y_idler_bracket (Autodesk Fusion 360 design; units mm, degrees)
Autodesk Fusion 360 part; units mm, degrees
sketch "Sketch1" plane through (0, 0, 0) normal (0, 0, 1) x (1, 0, 0)
  line L0 (0, 13) -> (0, -13) construction
  circle A0 centre (0, 13) radius 1.7
  circle A1 centre (0, -13) radius 1.7
  line L1 (-15, 14.35) -> (15, 14.35)
  line L2 (15, 14.35) -> (15, -21.5)
  line L3 (15, -21.5) -> (-15, -21.5)
  line L4 (-15, -21.5) -> (-15, 14.35)
  line L5 (-15, 19.35) -> (15, 19.35)
  line L6 (15, 19.35) -> (15, 14.35)
  line L7 (-15, 14.35) -> (-15, 19.35)
  line L8 (-15, -18.5) -> (-12, -21.5)
  line L9 (15, -18.5) -> (12, -21.5)
  line L10 (15, 17) -> (-15, 17)
  line L11 (-0.7632, 11.3) -> (0.7632, 11.3)
  line L12 (-1.2042, 11.8) -> (1.2042, 11.8)
  line L13 (1.2704, 11.8704) -> (0.7632, 11.3)
  line L14 (-1.2704, 11.8704) -> (-0.7632, 11.3)
  line L15 (-0.7042, -14.7) -> (0.7042, -14.7)
  line L16 (1.2021, -14.2021) -> (0.7042, -14.7)
  line L17 (0, -13) -> (1.2021, -14.2021) construction
  line L18 (0, -13) -> (-1.2021, -14.2021) construction
  line L19 (-1.2021, -14.2021) -> (-0.7042, -14.7)
  circle A2 centre (0, -13) radius 2.25
  line L20 (-1.591, -14.591) -> (-0.932, -15.25)
  line L21 (1.591, -14.591) -> (0.932, -15.25)
  line L22 (0.932, -15.25) -> (-0.932, -15.25)
  line L23 (-1.4142, -14.75) -> (1.4142, -14.75)
  line L24 (-1.2042, -14.2) -> (1.2042, -14.2) construction
  circle A3 centre (0, 13) radius 2.25
  line L25 (1.0102, 10.75) -> (-1.0102, 10.75)
  line L26 (-1.6814, 11.5049) -> (-1.0102, 10.75)
  line L27 (1.6814, 11.5049) -> (1.0102, 10.75)
  point P0 (0, -13)
  point P1 (0, 13)
  point P2 (0, -15.25)
  point P3 (0, 10.75)
  dimension "d1" = 26
  dimension "d2" = 3.4
  dimension "d3" = 3.4
  dimension "d4" = 30
  dimension "d6" = 8.5
  dimension "d7" = 15
  dimension "d8" = 5
  dimension "d10" = 45
  dimension "d11" = 3
  dimension "d38" = 40.85
  dimension "d60" = 2.35
  dimension "d74" = 0.5
  dimension "d81" = 4.5
  dimension "d82" = 0.5
  dimension "d83" = 0.5
  dimension "d84" = 135
  dimension "d90" = 4.5
  constraint vertical L0
  constraint coincident L0.start A0.centre
  constraint midpoint origin L0
  constraint coincident P0 L0.end
  constraint horizontal L1
  constraint vertical L2
  constraint horizontal L3
  constraint vertical L4
  constraint horizontal L5
  constraint vertical L6
  constraint vertical L7
  constraint coincident L1.start L4.end
  constraint coincident L1.end L2.start
  constraint coincident L4 L8.start
  constraint coincident L3 L8.end
  constraint symmetric L0 L8.start L9.start
  constraint symmetric L0 L8.end L9.end
  constraint coincident P1 L0.start
  constraint coincident L6 L10.start
  constraint coincident L7 L10.end
  constraint horizontal L10
  constraint horizontal L11
  constraint tangent A0 L11
  constraint coincident A0 L12.start
  constraint coincident A0 L12.end
  constraint horizontal L12
  constraint coincident A0 L13.start
  constraint tangent A0 L13
  constraint coincident L11.end L13.end
  constraint coincident A0 L14.start
  constraint tangent A0 L14
  constraint coincident L11.start L14.end
  constraint horizontal L15
  constraint tangent A1 L15
  constraint coincident A1 L16.start
  constraint tangent A1 L16
  constraint coincident L15.end L16.end
  constraint perpendicular L16 L17
  constraint coincident L16.start L17.end
  constraint perpendicular L17 L18
  constraint coincident A1 L18.end
  constraint tangent A1 L19
  constraint coincident L15.start L19.end
  constraint perpendicular L18 L19
  constraint coincident A2 L20.start
  constraint tangent A2 L20
  constraint coincident A2 L21.start
  constraint tangent A2 L21
  constraint horizontal L22
  constraint coincident L20.end L22.end
  constraint tangent A2 L22
  constraint coincident A2 L23.start
  constraint coincident A2 L23.end
  constraint horizontal L23
  constraint coincident A1 L24.start
  constraint coincident A1 L24.end
  constraint horizontal L24
  constraint coincident A2 P2
  constraint coincident L0 P2
  constraint midpoint L22 P2
  constraint parallel L19 L20
  constraint concentric A0 A3
  constraint horizontal L25
  constraint coincident A3 P3
  constraint coincident L0 P3
  constraint midpoint L25 P3
  constraint coincident A3 L26.start
  constraint tangent A3 L26
  constraint coincident A3 L27.start
  constraint tangent A3 L27
  constraint coincident L25.start L27.end
  constraint coincident L25.end L26.end
  constraint parallel L14 L26
  constraint parallel L13 L27
  measures "d1" distance of L0.start P0
  measures "d2" diameter of A0
  measures "d3" diameter of A1
  measures "d4" distance of L1.start L1.end
  measures "d6" distance of P0 L3
  measures "d7" distance of P0 L2
  measures "d8" distance of L5.end L1.end
  measures "d10" angle of L3 L8
  measures "d11" distance of L3.end L8.end
  measures "d38" distance of L3.end L5.start
  measures "d60" distance of L5.end L10.start
  measures "d74" distance of L11 L12
  measures "d81" diameter of A2
  measures "d82" distance of L22 L23
  measures "d83" distance of L15 L24
  measures "d84" angle of L0 L17
  measures "d90" diameter of A3
extrude "Extrude1" add sketch "Sketch1" along normal blind 11.8 contours A0 L1 L12 | A0 L1 L11 L13 L14 A3 | A0 L11 L14 | A0 L12 | A0 L1 A3 | A0 L1 | A0 L11 L13 | L1 L2 L3 L4 L8 L9 A3 L25 L26 L27 | L1 L6 L7 L10 A3 | A3 L25 L26 | L5 L6 L7 L10 | A3 L25 L27 | A1 | A1 L15 L19 | A1 L15 L16 | A2 L23 | A2 L20 L22 | A2 L21 L22 | A2 L23
extrude "Extrude2" add sketch "Sketch1" along normal blind 54.6 contours A0 L1 A3 | A0 L1 | L1 L6 L7 L10 A3 | L5 L6 L7 L10
sketch "Sketch2" plane through (0, 14.35, 0) normal (0, -1, 0) x (1, 0, 0)
  line L0 (-15, 11.8) -> (15, 11.8)
  line L1 (15, 11.8) -> (15, 54.6)
  line L2 (15, 54.6) -> (-15, 54.6)
  line L3 (-15, 54.6) -> (-15, 11.8)
  circle A0 centre (0, 40) radius 1.6
  circle A1 centre (0, 40) radius 2.25
  dimension "d16" = 30
  dimension "d17" = 42.8
  dimension "d18" = 3.2
  dimension "d19" = 15
  dimension "d20" = 14.6
  dimension "d76" = 4.5
  constraint concentric A0 A1
  measures "d16" distance of L1.end L2.end
  measures "d17" distance of L0.end L1.end
  measures "d18" diameter of A0
  measures "d19" horizontal distance of L1.end A0.centre
  measures "d20" vertical distance of L1.end A0.centre
  measures "d76" diameter of A1
extrude "Extrude3" cut sketch "Sketch2" against normal blind 13 contours A0
extrude "Extrude6" cut sketch "Sketch1" along normal blind 6.8 contours A0 L1 L12 | A0 L11 L14 | A0 L12 | A0 L1 | A0 L11 L13 | A1 | A1 L15 L19 | A1 L15 L16
extrude "Extrude9" add sketch "Sketch1" against normal blind 4.2 contours L5 L6 L7 L10
extrude "Extrude11" cut sketch "Sketch2" against normal blind 5 contours A0 | A1
chamfer "Chamfer16" distance 0.625 angle 45 1 edges at (-2.0977, 19.35, 39.1864)
sketch "Sketch5" plane through (-15, 0, 0) normal (-1, 0, 0) x (0, -1, 0)
  line L0 (-17, 0) -> (18.5, 0)
  line L1 (18.5, 0) -> (18.5, 11.8)
  line L2 (18.5, 11.8) -> (-14.35, 11.8)
  line L3 (-14.35, 11.8) -> (-14.35, 54.6)
  line L4 (-14.35, 54.6) -> (-19.35, 54.6)
  line L5 (-19.35, 54.6) -> (-19.35, -4.2)
  line L6 (-19.35, -4.2) -> (-17, -4.2)
  line L7 (-17, -4.2) -> (-17, 0)
  circle A0 centre (-17, 0) radius 0.5
  dimension "d63" = 1
  constraint coincident L0.start L7.end
  measures "d63" diameter of A0
extrude "Extrude10" cut sketch "Sketch5" against normal blind 30 contours L0 L7 A0 | L0 L7 A0
chamfer "Chamfer1" distance 3 angle 45 2 edges at (15, 16.85, 54.6) (-15, 16.85, 54.6)
chamfer "Chamfer11" distance 20 angle 45 1 edges at (0, 14.35, 11.8)
chamfer "Chamfer2" distance 1 angle 45 12 edges at (-15, 14.35, 41.7) (-13.5, 14.35, 53.1) (0, 14.35, 54.6) (13.5, 14.35, 53.1) (15, 14.35, 41.7) (15, -12.075, 11.8) (13.5, -20, 11.8) (0, -21.5, 11.8) (-13.5, -20, 11.8) (-15, -12.075, 11.8) (-15, 4.35, 21.8) (15, 4.35, 21.8)
fillet "Fillet2" radius 2 2 edges at (-15, 18.175, -4.2) (15, 18.175, -4.2)
fillet "Fillet3" radius 0.5 2 edges at (0, 17, -0.5) (0, 16.5, 0)
chamfer "Chamfer14" distance 0.4 angle 45 16 edges at (15, -1.183, 0) (15, 16.384, 0.067) (15, 17.3536, 0.3536) (15, 17.067, -0.616) (15, 17, -1.533) (14.4142, 17, -3.6142) (0, 17, -4.2) (-14.4142, 17, -3.6142) (-15, 17, -1.533) (-15, 17.067, -0.616) (-15, 17.3536, 0.3536) (-15, 16.384, 0.067) (-15, -1.183, 0) (13.5, -20, 0) (0, -21.5, 0) (-13.5, -20, 0)
chamfer "Chamfer15" distance 0.4 angle 45 8 edges at (-15, 19.35, 24.7) (-14.4142, 19.35, -3.6142) (0, 19.35, -4.2) (14.4142, 19.35, -3.6142) (15, 19.35, 24.7) (-13.5, 19.35, 53.1) (0, 19.35, 54.6) (13.5, 19.35, 53.1)
chamfer "Chamfer17" distance 0.4 angle 45 1 edges at (-2.0977, 14.35, 40.8136)
extrude "Extrude13" cut sketch "Sketch1" along normal blind 5 contours A0 L1 L11 L13 L14 A3 | A0 L11 L14 | A0 L12 | A0 L1 A3 | A0 L11 L13 | A3 L25 L26 | A3 L25 L27 | A1 | A1 L15 L19 | A1 L15 L16 | A2 L23 | A2 L20 L22 | A2 L21 L22 | A2 L23
chamfer "Chamfer20" distance 0.525 angle 45 8 edges at (1.0168, 11.5852, 5) (0, 14.7, 5) (-1.0168, 11.5852, 5) (0, 11.3, 5) (0, -11.3, 5) (0.9531, -14.451, 5) (-0.9531, -14.451, 5) (0, -14.7, 5)
chamfer "Chamfer21" distance 0.4 angle 45 6 edges at (1.3458, 11.1274, 0) (0, 15.25, 0) (-1.3458, 11.1274, 0) (0, -10.75, 0) (-1.2615, -14.9205, 0) (1.2615, -14.9205, 0)
move_body "Move1" bodies 1 to x (-1, 0, 0) y (0, 0, -1) z (0, -1, 0) at (-30, -21.5, -21.5)
move_body "Move2" bodies 1 to x (1, 0, 0) y (0, 1, 0) z (0, 0, 1) at (30, 46.7, 40.85)
equation "d3 = d2"
equation "d7 = d4 / 2"
equation "d14 = 38 mm + 10 mm + 6.6 mm"
equation "d19 = d16 / 2"
equation "d20 = 8 mm + 6.6 mm"
equation "d38 = 38.5 mm + 2.35 mm"
equation "d42 = 11 mm - 4.2 mm"
